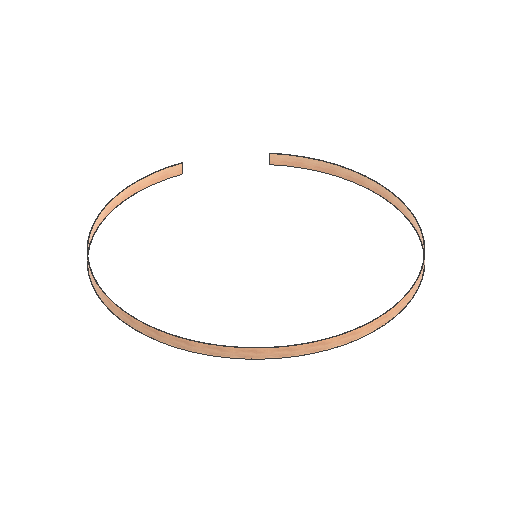
# Autodesk Inventor part: Edge Band - Platform C Outer
Saved by Autodesk Inventor 2021 (Build 250183000, 183)
## iProperties
Created: 2020-05-12
Part Number: Edge Band - Platform C Outer
Material: Wood (Birch)
Document SubType Name: Modeling
Designer: Dan Wikman
Density: 0.55 g/cm^3
Appearance: Birch - Natural Polished
Mass: 1544.61 g
Surface Area: 14611.7 cm^2
Volume: 2808.39 cm^3
Author: Dan Wikman
Autodesk Inventor part; units mm, degrees
ref_plane "YZ Plane" through (0, 0, 0) normal (1, 0, 0) x (0, 1, 0)
ref_plane "XZ Plane" through (0, 0, 0) normal (0, 1, 0) x (-1, 0, 0)
ref_plane "XY Plane" through (0, 0, 0) normal (0, 0, 1) x (1, 0, 0)
sketch "Sketch1" plane through (0, 0, 0) normal (0, 1, 0) x (-1, 0, 0)
  circle A0 centre (0, 0) radius 1218.81
  circle A1 centre (0, 0) radius 1222.81
  dimension "d0" = 2437.62
  dimension "d1" = 2445.62
  constraints: 2 centre point, 2 coincident
  measures "d0" diameter of A0
  measures "d1" diameter of A1
extrude "Extrusion1" add sketch "Sketch1" along normal blind 100
sketch "Sketch2" plane through (0, 0, 0) normal (0, -1, 0) x (1, 0, 0)
  line L0 (-1152.0758, -397.7746) -> (-847.4557, -240.1463) projected
  line L1 (-532.6414, -700.6187) -> (-790.0726, -927.2533) projected
  circle A0 centre (0, 0) radius 1222.81 projected
  line L2 (-793.5677, -930.3303) -> (-790.5345, -927.66)
  circle A1 centre (0, 0) radius 1218.81 projected
  line L3 (-1156.7304, -400.1831) -> (-1151.0362, -397.2366)
  point P0 (-1155.6639, -399.6313)
  point P1 (-1152.0738, -397.7735)
  constraints: 4 end point, 1 point on line, 4 other
extrude "Extrusion2" cut sketch "Sketch2" against normal blind 100 contours A0 L3 A1 L2 picked at (-803.1153, -918.3043)
body "Solid1"
